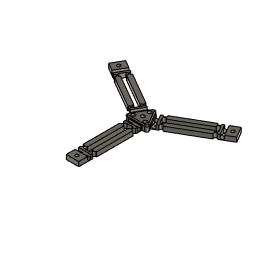
soft_delta (Autodesk Fusion 360 design; units mm, degrees)
Autodesk Fusion 360 part; units mm, degrees
sketch "Sketch1" plane through (0, 0, 0) normal (0, 0, 1) x (1, 0, 0)
  line L0 (0, 0) -> (0, -7.2169) construction
  line L1 (-12.5, -7.2169) -> (12.5, -7.2169)
  line L2 (12.5, -7.2169) -> (0, 14.4338)
  line L3 (0, 14.4338) -> (-12.5, -7.2169)
  line L4 (0, 0) -> (6.25, 3.6084) construction
  line L5 (0, 0) -> (-6.25, 3.6084) construction
  dimension "d1" = 25
  constraint coincident L0.start L4.start
  constraint vertical L0
  constraint perpendicular L0 L1
  constraint equal L1 L2
  constraint equal L2 L3
  constraint coincident L2 L4.end
  constraint perpendicular L2 L4
  constraint coincident L3 L5.end
  constraint perpendicular L3 L5
  constraint equal L0 L4
  constraint equal L4 L5
  constraint coincident L0.end L1
  measures "d1" distance of L1.start L2.end
extrude "Extrude1" add sketch "Sketch1" along normal blind 5.5 makes body 1
fillet "Fillet1" radius 2 3 edges at (-12.5, -7.2169, 2.75) (12.5, -7.2169, 2.75) (0, 14.4338, 2.75) on bodies 1
fillet "Fillet2" radius 1 1 faces at (0.5774, 1, 5.5) on bodies 1
sketch "Sketch2" plane through (0, -7.2169, 0) normal (0, -1, 0) x (1, 0, 0)
  line L0 (9.0359, 4.5) -> (-9.0359, 4.5)
  line L1 (-9.0359, 4.5) -> (-9.0359, 0)
  line L2 (-9.0359, 0) -> (9.0359, 0)
  line L3 (9.0359, 0) -> (9.0359, 4.5)
  line L4 (-6.3, 4.5) -> (6.3, 4.5)
  line L5 (6.3, 4.5) -> (6.3, 0)
  line L6 (6.3, 0) -> (-6.3, 0)
  line L7 (-6.3, 0) -> (-6.3, 4.5)
  point P0 (0, 4.5)
  dimension "d8" = 12.6
  constraint horizontal L4
  constraint vertical L5
  constraint horizontal L6
  constraint vertical L7
  constraint coincident L2 L5.end
  constraint coincident L0 L4.start
  constraint midpoint L4 P0
  constraint vertical origin P0
  measures "d8" distance of L5 L7
extrude "Extrude2" add sketch "Sketch2" along normal blind 6.25 contours L0 L2 L4 L5 L6 L7 bodies 1
sketch "Sketch3" plane through (-6.3, 0, 0) normal (-1, 0, 0) x (0, -1, 0)
  line L0 (7.2169, 4.5) -> (7.2169, 0)
  line L1 (7.2169, 0) -> (13.4669, 0)
  line L2 (13.4669, 0) -> (13.4669, 4.5)
  line L3 (13.4669, 4.5) -> (7.2169, 4.5)
sketch "Sketch4" plane through (-6.3, -10.3419, 2.25) normal (-1, 0, 0) x (0, -1, 0)
  line L0 (-2.125, 2.25) -> (1.125, 2.25)
  line L1 (1.125, 2.25) -> (1.125, -0.215)
  line L2 (-2.125, 2.25) -> (-2.125, -0.215)
  arc A0 (-2.125, -0.215) -> (1.125, -0.215) centre (-0.5, -0.215) ccw
  line L3 (3.125, 2.25) -> (-3.125, 2.25)
  line L4 (-2.125, -1.84) -> (1.125, -1.84) construction
  line L5 (-3.125, -2.25) -> (3.125, -2.25)
  point P0 (-3.125, 2.25)
  point P1 (3.125, 2.25)
  dimension "d13" = 0.41
  dimension "d15" = 1
  dimension "d16" = 2
  constraint horizontal L0
  constraint perpendicular L0 L1
  constraint perpendicular L0 L2
  constraint tangent L2 A0
  constraint tangent L1 A0
  constraint collinear L0 L3
  constraint coincident L0.end L3
  constraint horizontal L4
  constraint vertical L0.end L4.end
  constraint vertical L0.start L4.start
  constraint tangent A0 L4
  measures "d13" distance of L4 L5
  measures "d15" distance of L0.start P0
  measures "d16" distance of L0.end P1
extrude "Extrude3" cut sketch "Sketch4" against normal up to surface (12.6 mm away) bodies 1
sketch "Sketch5" plane through (0, 0, 4.5) normal (0, 0, 1) x (-1, 0, 0)
  line L0 (-6.3, 11.4669) -> (6.3, 11.4669)
  line L1 (6.3, 11.4669) -> (6.3, 13.4669)
  line L2 (6.3, 13.4669) -> (-6.3, 13.4669)
  line L3 (-6.3, 13.4669) -> (-6.3, 11.4669)
  arc A0 (6.3, 16.7169) -> (6.3, 13.4669) centre (6.3, 15.0919) ccw
  arc A1 (2.64, 13.4669) -> (2.64, 16.7169) centre (2.64, 15.0919) ccw
  line L4 (4.265, 18) -> (4.265, 15.0919) construction
  line L5 (4.675, 18) -> (4.675, 15.0919) construction
  line L6 (2.22, 16.7169) -> (2.22, 53.7169)
  line L7 (6.72, 53.7169) -> (6.72, 16.7169)
  line L8 (2.64, 13.4669) -> (6.3, 13.4669)
  line L9 (6.72, 16.7169) -> (6.3, 16.7169)
  line L10 (2.64, 16.7169) -> (2.22, 16.7169)
  line L11 (2.22, 35.2169) -> (6.72, 35.2169) construction
  arc A2 (6.3, 56.9669) -> (6.3, 53.7169) centre (6.3, 55.3419) ccw
  arc A3 (2.64, 53.7169) -> (2.64, 56.9669) centre (2.64, 55.3419) ccw
  line L12 (2.64, 56.9669) -> (6.3, 56.9669)
  line L13 (6.72, 53.7169) -> (6.3, 53.7169)
  line L14 (2.64, 53.7169) -> (2.22, 53.7169)
  dimension "d19" = 1.625
  dimension "d20" = 0.41
  dimension "d21" = 4.5
  dimension "d23" = 37
  constraint coincident L1.end L2.start
  constraint tangent L2 A0
  constraint vertical L1.end A0.start
  constraint equal A0 A1
  constraint vertical A1.start A1.end
  constraint tangent L2 A1
  constraint coincident L2 A1.start
  constraint vertical L4
  constraint tangent A1 L4
  constraint coincident A0 L5.end
  constraint vertical L5
  constraint tangent A0 L5
  constraint midpoint A1 L4.end
  constraint horizontal L9
  constraint vertical L6
  constraint vertical L7
  constraint collinear L9 L10
  constraint equal L9 L10
  constraint midpoint L6 L11.start
  constraint midpoint L7 L11.end
  constraint symmetric L1.end L11 A2.start
  constraint symmetric A0.start L11 A2.end
  constraint symmetric A0 L11 A2
  constraint symmetric A1.start L11 A3.end
  constraint symmetric A1.end L11 A3.start
  constraint symmetric A1 L11 A3
  constraint symmetric L7.end L11 L7.start
  constraint symmetric L6.start L11 L6.end
  constraint horizontal L6.end L7.start
  measures "d16" distance of L5.start
  measures "d19" radius of A0
  measures "d20" distance of L4 L5
  measures "d21" distance of L6.end L7.start
  measures "d23" vertical distance of A0.start L7.start
extrude "Extrude4" add sketch "Sketch5" against normal up to surface (4.5 mm away) separate body contours L2 A0 A1 L6 L7 L8 L9 L10 A2 A3 L12 L13 L14 makes body 2
ref_plane "WorkPlane1" through (0, -10.3419, 2.25) normal (1, 0, 0) x (0, 0, 1)
mirror "Mirror1" about plane through (0, -10.3419, 2.25) normal (1, 0, 0) of bodies 2 makes body 3
combine "Combine1" operation add target body 1 tool bodies 2 3
sketch "Sketch8" plane through (0, 0, 0) normal (0, 0, -1) x (1, 0, 0)
  arc A0 (-1.7321, -11.4338) -> (1.7321, -11.4338) centre (0, -10.4338) ccw
  line L0 (1.7321, -11.4338) -> (10.7679, 4.2169)
  arc A1 (10.7679, 4.2169) -> (9.0359, 7.2169) centre (9.0359, 5.2169) ccw
  line L1 (9.0359, 7.2169) -> (6.3, 7.2169)
  line L2 (6.3, 7.2169) -> (6.3, 13.4669)
  arc A2 (6.3, 16.7169) -> (6.3, 13.4669) centre (6.3, 15.0919) ccw
  line L3 (6.3, 16.7169) -> (6.72, 16.7169)
  line L4 (6.72, 16.7169) -> (6.72, 53.7169)
  line L5 (6.72, 53.7169) -> (6.3, 53.7169)
  arc A3 (6.3, 56.9669) -> (6.3, 53.7169) centre (6.3, 55.3419) ccw
  line L6 (6.3, 56.9669) -> (2.64, 56.9669)
  arc A4 (2.64, 53.7169) -> (2.64, 56.9669) centre (2.64, 55.3419) ccw
  line L7 (2.64, 53.7169) -> (2.22, 53.7169)
  line L8 (2.22, 53.7169) -> (2.22, 16.7169)
  line L9 (2.22, 16.7169) -> (2.64, 16.7169)
  arc A5 (2.64, 13.4669) -> (2.64, 16.7169) centre (2.64, 15.0919) ccw
  line L10 (2.64, 13.4669) -> (-2.64, 13.4669)
  arc A6 (-2.64, 16.7169) -> (-2.64, 13.4669) centre (-2.64, 15.0919) ccw
  line L11 (-2.64, 16.7169) -> (-2.22, 16.7169)
  line L12 (-2.22, 16.7169) -> (-2.22, 53.7169)
  line L13 (-2.22, 53.7169) -> (-2.64, 53.7169)
  arc A7 (-2.64, 56.9669) -> (-2.64, 53.7169) centre (-2.64, 55.3419) ccw
  line L14 (-2.64, 56.9669) -> (-6.3, 56.9669)
  arc A8 (-6.3, 53.7169) -> (-6.3, 56.9669) centre (-6.3, 55.3419) ccw
  line L15 (-6.3, 53.7169) -> (-6.72, 53.7169)
  line L16 (-6.72, 53.7169) -> (-6.72, 16.7169)
  line L17 (-6.72, 16.7169) -> (-6.3, 16.7169)
  arc A9 (-6.3, 13.4669) -> (-6.3, 16.7169) centre (-6.3, 15.0919) ccw
  line L18 (-6.3, 13.4669) -> (-6.3, 7.2169)
  line L19 (-6.3, 7.2169) -> (-9.0359, 7.2169)
  arc A10 (-9.0359, 7.2169) -> (-10.7679, 4.2169) centre (-9.0359, 5.2169) ccw
  line L20 (-10.7679, 4.2169) -> (-1.7321, -11.4338)
  line L21 (-6.3, 56.9669) -> (6.3, 56.9669)
  line L22 (6.3, 56.9669) -> (6.3, 71.2169)
  line L23 (6.3, 71.2169) -> (-6.3, 71.2169)
  line L24 (-6.3, 71.2169) -> (-6.3, 56.9669)
  dimension "d32" = 14.25
  constraint horizontal L21
  constraint vertical L22
  constraint horizontal L23
  constraint vertical L24
  constraint coincident L14.end A8.end
  measures "d32" distance of A3.start L22.end
extrude "Extrude6" add sketch "Sketch8" against normal up to surface (4.5 mm away) contours L6 L14 L21 L22 L23 L24 bodies 1
ref_plane "WorkPlane2" through (-6.51, -35.2169, 2.25) normal (0, 1, 0) x (1, 0, 0)
sketch "Sketch10" plane through (0, 0, 4.5) normal (0, 0, 1) x (-1, 0, 0)
  arc A0 (-6.3, 53.7169) -> (-6.3, 56.9669) centre (-6.3, 55.3419) ccw
  line L0 (-6.3, 53.7169) -> (-6.72, 53.7169)
  line L1 (-6.72, 53.7169) -> (-6.72, 16.7169)
  line L2 (-6.72, 16.7169) -> (-6.3, 16.7169)
  arc A1 (-6.3, 13.4669) -> (-6.3, 16.7169) centre (-6.3, 15.0919) ccw
  line L3 (-6.3, 13.4669) -> (-6.3, 11.4669)
  line L4 (-6.3, 11.4669) -> (6.3, 11.4669)
  line L5 (6.3, 11.4669) -> (6.3, 13.4669)
  arc A2 (6.3, 16.7169) -> (6.3, 13.4669) centre (6.3, 15.0919) ccw
  line L6 (6.3, 16.7169) -> (6.72, 16.7169)
  line L7 (6.72, 16.7169) -> (6.72, 53.7169)
  line L8 (6.72, 53.7169) -> (6.3, 53.7169)
  arc A3 (6.3, 56.9669) -> (6.3, 53.7169) centre (6.3, 55.3419) ccw
  line L9 (6.3, 56.9669) -> (6.3, 71.2169)
  line L10 (6.3, 71.2169) -> (-6.3, 71.2169)
  line L11 (-6.3, 71.2169) -> (-6.3, 56.9669)
  line L12 (-2.64, 56.9669) -> (2.64, 56.9669)
  arc A4 (2.64, 53.7169) -> (2.64, 56.9669) centre (2.64, 55.3419) ccw
  line L13 (2.64, 53.7169) -> (2.22, 53.7169)
  line L14 (2.22, 53.7169) -> (2.22, 16.7169)
  line L15 (2.22, 16.7169) -> (2.64, 16.7169)
  arc A5 (2.64, 13.4669) -> (2.64, 16.7169) centre (2.64, 15.0919) ccw
  line L16 (2.64, 13.4669) -> (-2.64, 13.4669)
  arc A6 (-2.64, 16.7169) -> (-2.64, 13.4669) centre (-2.64, 15.0919) ccw
  line L17 (-2.64, 16.7169) -> (-2.22, 16.7169)
  line L18 (-2.22, 16.7169) -> (-2.22, 53.7169)
  line L19 (-2.22, 53.7169) -> (-2.64, 53.7169)
  arc A7 (-2.64, 56.9669) -> (-2.64, 53.7169) centre (-2.64, 55.3419) ccw
  line L20 (1.8, 8.2169) -> (-1.8, 8.2169)
  line L21 (-1.8, 8.2169) -> (-1.8, 11.4669)
  line L22 (-1.8, 11.4669) -> (1.8, 11.4669)
  line L23 (1.8, 11.4669) -> (1.8, 8.2169)
  line L24 (6.3, 8.2169) -> (-6.3, 8.2169)
  line L25 (6.3, 13.4669) -> (6.3, 7.2169)
  line L26 (-6.3, 8.2169) -> (-6.3, 11.4669)
  dimension "d38" = 4.5
  dimension "d39" = 4.5
  constraint horizontal L20
  constraint vertical L21
  constraint horizontal L22
  constraint vertical L23
  constraint coincident L4 L21.end
  constraint collinear L20 L24
  constraint coincident L20.start L24
  measures "d38" distance of L23 L25
  measures "d39" distance of L21.end L26
extrude "Extrude7" cut sketch "Sketch10" against normal up to surface (4.5 mm away) contours L4 L20 L21 L22 L23 L24 bodies 1
mirror "Mirror2" about plane through (-6.51, -35.2169, 2.25) normal (0, 1, 0) of "Extrude3", "Extrude7"
ref_plane "WorkPlane3" through (-7.6679, -7.2169, 2.25) normal (0, -1, 0) x (1, 0, 0)
split "Split1" by plane through (-7.6679, -7.2169, 2.25) normal (0, -1, 0) bodies 1 makes body 4 at (-0.6, -68.2169, 0)
sketch "Sketch11" plane through (0, 0, 4.5) normal (0, 0, 1) x (-1, 0, 0)
  line L0 (-6.3, 62.2169) -> (6.3, 62.2169)
  line L1 (6.3, 62.2169) -> (6.3, 71.2169)
  line L2 (6.3, 71.2169) -> (-6.3, 71.2169)
  line L3 (-6.3, 71.2169) -> (-6.3, 62.2169)
  line L4 (6.3, 62.2169) -> (-6.3, 71.2169) construction
  circle A0 centre (0, 66.7169) radius 1.65
  dimension "d42" = 3.3
  constraint coincident L0.end L1.start
  constraint coincident L2.end L3.start
  constraint midpoint L4 A0.centre
  measures "d42" diameter of A0
extrude "Extrude8" cut sketch "Sketch11" against normal up to surface (4.5 mm away) contours A0 bodies 4
pattern_circular "C-Pattern1" count 3 over 360 about axis through (0, 0, 1.75) along (0, 0, 1) of bodies 4 makes body 5 at (57.3639, 27.5765, 0) makes body 6 at (-52.5639, 35.8904, 0)
combine "Combine2" operation add target body 1 tool bodies 4 5 6
sketch "Sketch12" plane through (0, 0, 5.5) normal (0, 0, 1) x (-1, 0, 0)
  arc A0 (-0.866, -10.9338) -> (0.866, -10.9338) centre (0, -10.4338) ccw
  line L0 (0.866, -10.9338) -> (9.9019, 4.7169)
  arc A1 (9.9019, 4.7169) -> (9.0359, 6.2169) centre (9.0359, 5.2169) ccw
  line L1 (9.0359, 6.2169) -> (-9.0359, 6.2169)
  arc A2 (-9.0359, 6.2169) -> (-9.9019, 4.7169) centre (-9.0359, 5.2169) ccw
  line L2 (-9.9019, 4.7169) -> (-0.866, -10.9338)
  circle A3 centre (0, 0) radius 3.84
  dimension "d45" = 7.68
  constraint coincident A3.centre origin
  measures "d45" diameter of A3
sketch "Sketch13" plane through (0, 0, 5.5) normal (0, 0, 1) x (-1, 0, 0)
  arc A0 (-0.866, -10.9338) -> (0.866, -10.9338) centre (0, -10.4338) ccw
  line L0 (0.866, -10.9338) -> (9.9019, 4.7169)
  arc A1 (9.9019, 4.7169) -> (9.0359, 6.2169) centre (9.0359, 5.2169) ccw
  line L1 (9.0359, 6.2169) -> (-9.0359, 6.2169)
  arc A2 (-9.0359, 6.2169) -> (-9.9019, 4.7169) centre (-9.0359, 5.2169) ccw
  line L2 (-9.9019, 4.7169) -> (-0.866, -10.9338)
  circle A3 centre (0, 0) radius 1.85
  circle A4 centre (0, -7) radius 1.85
  circle A5 centre (6.0622, 3.5) radius 1.85
  circle A6 centre (-6.0622, 3.5) radius 1.85
  line L3 (9.9019, 5.7169) -> (0, 0) construction
  line L4 (0, 0) -> (-9.9019, 5.7169) construction
  dimension "d48" = 3.7
  dimension "d49" = 7
  dimension "d50" = 7
  dimension "d51" = 7
  constraint coincident A3.centre L3.end
  constraint equal A3 A4
  constraint equal A4 A6
  constraint equal A3 A5
  constraint vertical A3.centre A4.centre
  constraint midpoint A1 L3.start
  constraint midpoint A2 L4.end
  constraint coincident A5.centre L3
  constraint coincident A6.centre L4
  measures "d48" diameter of A3
  measures "d49" distance of A3.centre A6.centre
  measures "d50" distance of A3.centre A5.centre
  measures "d51" distance of A3.centre A4.centre
extrude "Extrude10" cut sketch "Sketch13" against normal blind 5.5 contours A3 | A4 | A5 | A6 bodies 1
sketch "Sketch14" plane through (0, 0, 5.5) normal (0, 0, 1) x (-1, 0, 0)
  arc A0 (-0.866, -10.9338) -> (0.866, -10.9338) centre (0, -10.4338) ccw
  line L0 (0.866, -10.9338) -> (9.9019, 4.7169)
  arc A1 (9.9019, 4.7169) -> (9.0359, 6.2169) centre (9.0359, 5.2169) ccw
  line L1 (9.0359, 6.2169) -> (-9.0359, 6.2169)
  arc A2 (-9.0359, 6.2169) -> (-9.9019, 4.7169) centre (-9.0359, 5.2169) ccw
  line L2 (-9.9019, 4.7169) -> (-0.866, -10.9338)
  line L3 (6.72, 8.2169) -> (-6.72, 8.2169)
  line L4 (-6.72, 8.2169) -> (-6.72, 71.2169)
  line L5 (-6.72, 71.2169) -> (6.72, 71.2169)
  line L6 (6.72, 71.2169) -> (6.72, 8.2169)
  line L7 (6.3, 8.2169) -> (-6.3, 8.2169)
  line L8 (-6.3, 71.2169) -> (6.3, 71.2169)
  line L9 (-6.72, 53.7169) -> (-6.72, 16.7169)
  line L10 (6.72, 53.7169) -> (6.72, 16.7169)
  circle A3 centre (0, 0) radius 1.85
  circle A4 centre (-6.0622, 3.5) radius 1.85
  circle A5 centre (0, -7) radius 1.85
  circle A6 centre (6.0622, 3.5) radius 1.85
  constraint horizontal L3
  constraint vertical L4
  constraint horizontal L5
  constraint vertical L6
  constraint collinear L3 L7
  constraint collinear L5 L8
  constraint collinear L4 L9
  constraint collinear L6 L10
extrude "Extrude12" add 1 faces at (-0.0461, -3.4834, 5.5) along direction (0, 0, 1) blind 3 separate body on bodies 1 makes body 7
copy_body "Body->Comp1" bodies 7 removing the originals makes body 8 in component "Component"
extrude "Extrude9" [suppressed]
component "Component" placed x (1, 0, 0) y (0, 1, 0) z (0, 0, 1) at (0, 0, 0)
